douillestator (Autodesk Fusion 360 design; units mm, degrees)
Autodesk Fusion 360 part; units mm, degrees
sketch "Esquisse1" plane through (0, 0, 0) normal (1, 0, 0) x (0, 1, 0)
  line L0 (0, 0) -> (-16, 0)
  line L1 (-16, 0) -> (-16, 6.5037)
  line L2 (-16, 6.5037) -> (-15.2163, 6.5037)
  line L3 (-15.2163, 6.5037) -> (-15.2163, 9.9566)
  line L4 (-15.2163, 9.9566) -> (-11.3366, 9.9566)
  line L5 (-11.3366, 9.9566) -> (-11.3366, 23)
  line L6 (-11.3366, 23) -> (0, 23)
  line L7 (0, 23) -> (0, 0)
  line L8 (0, 2.5) -> (0, 20)
  dimension "d1" = 16
  dimension "d2" = 15.2163
  constraint coincident L0.start L7.end
  constraint horizontal L0
  constraint perpendicular L0 L1
  constraint perpendicular L1 L2
  constraint perpendicular L2 L3
  constraint perpendicular L2 L5
  constraint perpendicular L5 L6
  constraint perpendicular L0 L7
  constraint horizontal L4
  measures "d1" distance of L0.start L0.end
  measures "d2" distance of L3 L8
revolve "Révolution1" add sketch "Esquisse1" angle 360 about axis through (0, 0, 23) along (0, 0, -1)
